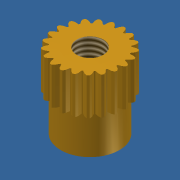
# Autodesk Inventor part: pinhon servo
Saved by Autodesk Inventor 2014 (Build 180170000, 170)
## iProperties
Created: 2010-09-11
Part Number: pinhon servo
Document SubType Name: Modeling
Designer: LEFO
Density: 1 g/cm^3
Material: Generic
Appearance: Brass - Satin
Author: LEFO
Autodesk Inventor part; units mm, degrees
ref_plane "YZ Plane" through (0, 0, 0) normal (1, 0, 0) x (0, 1, 0)
ref_plane "XZ Plane" through (0, 0, 0) normal (0, 1, 0) x (-1, 0, 0)
ref_plane "XY Plane" through (0, 0, 0) normal (0, 0, 1) x (1, 0, 0)
sketch "Sketch1" plane through (0, 0, 0) normal (0, 0, 1) x (1, 0, 0)
  circle A0 centre (-0.0131, 0.0043) radius 2.75
  line L0 (-0.2631, 3.0543) -> (-0.1131, 3.2543)
  line L1 (-0.1131, 3.2543) -> (0.0869, 3.2543)
  line L2 (0.0869, 3.2543) -> (0.2369, 3.0543)
  line L3 (-0.2631, 3.0543) -> (-0.37, 2.7311)
  line L4 (0.2369, 3.0543) -> (0.3439, 2.7311)
  line L5 (-0.0131, 3.2543) -> (-0.0131, 0.0043) construction
  line L6 (-0.37, 2.7311) -> (0.3439, 2.7311)
  circle A1 centre (-0.0131, 0.0043) radius 2.75
  circle A2 centre (-0.0131, 0.0043) radius 2.75
  dimension "d0" = 5.5
  dimension "d12" = 0.2
  dimension "d18" = 0.5
  dimension "d19" = 0.7139
  dimension "d23" = 0.3233
  dimension "d24" = 71.693
  dimension "d25" = 71.693
  dimension "d26" = 53.124
  constraints: 14 end point, 4 coincident, 2 point on circle, 1 centre point, 1 equal length, 1 midpoint, 1 perpendicular, 1 vertical, 6 other
  measures "d0" diameter of A0
  measures "d12" distance of L0.end L1.end
  measures "d18" distance of L2.end L0.start
  measures "d19" distance of L4.end L6.start
  measures "d23" distance from line of L6 L0.start
  measures "d24" angle of L6 L3
  measures "d25" angle of L6 L4
  measures "d26" angle of L6 L0
extrude "Extrusion1" add sketch "Sketch1" along normal blind 3.5 contours A0 L6 | L6 A0
extrude "Extrusion2" add sketch "Sketch1" along normal blind 3.5 contours A0 L3 L0 L1 L2 L4
pattern_circular "Circular Pattern1" count 21 over 360 about axis through (-0.0131, 0.0043, 0) along (0, 0, 1) of "Extrusion2"
sketch "Sketch3" plane through (0, 0, 0) normal (0, 0, -1) x (-1, 0, 0)
  arc A0 (0.4757, 2.7151) -> (0.37, 2.7311) centre (0.0131, 0.0043) ccw projected
  circle A1 centre (0.0131, 0.0043) radius 2.75
  dimension "d46" = 5.5
  constraints: 1 centre point, 1 coincident
  measures "d46" diameter of A1
extrude "Extrusion3" add sketch "Sketch3" along normal blind 3.5
hole "Hole1" at (-0.0131, 0.0043, 3.5) direction (0, 0, -1) diameter 2.5 depth 7
thread "Thread1" size "M2.5x0.45" class "6H" standard "ANSI Metric M Profile" full length
body "Solid1"
